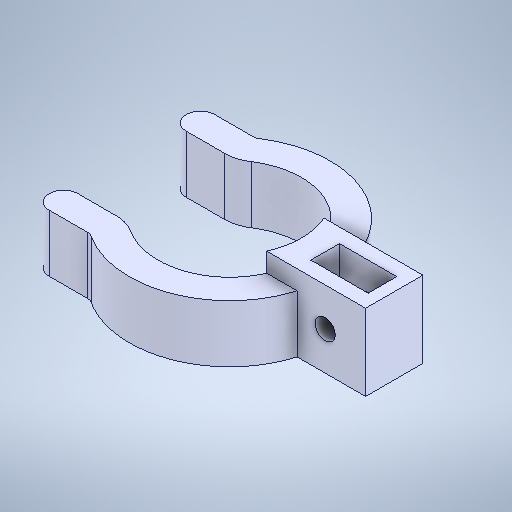
# Autodesk Inventor part: sujetador_marcador_v2
Saved by Autodesk Inventor 2025.2 (Build 292293000, 293)
## iProperties
Created: 2024-08-16
Part Number: sujetador_marcador_v2
Material: Generic
Document SubType Name: Modeling
Designer: cdavi
Density: 1 g/cm^3
Appearance: Default
Sending System: SolidWorks 2024
Last Author: jimen
Last Saved: 2024-10-09
Author: cdavi
Autodesk Inventor part; units mm, degrees
ref_plane "YZ Plane" through (0, 0, 0) normal (1, 0, 0) x (0, 1, 0)
ref_plane "XZ Plane" through (0, 0, 0) normal (0, 1, 0) x (-1, 0, 0)
ref_plane "XY Plane" through (0, 0, 0) normal (0, 0, 1) x (1, 0, 0)
sketch "Sketch1" plane through (0, 0, 0) normal (0, 1, 0) x (-1, 0, 0)
  circle A0 centre (0, 0) radius 7.5
  circle A1 centre (0, 0) radius 10.5
  line L0 (0, 0) -> (5.6818, 8.8299) construction
  line L1 (0, 0) -> (0, 10.5)
  line L2 (6.222, 8.6714) -> (10.222, 8.6714)
  arc A2 (5.6818, 8.8299) -> (6.222, 8.6714) centre (6.222, 9.6714) ccw
  line L3 (6.222, 5.6714) -> (10.222, 5.6714)
  arc A3 (4.0584, 6.3071) -> (6.222, 5.6714) centre (6.222, 9.6714) ccw
  line L4 (10.222, 8.6714) -> (10.222, 5.6714) construction
  arc A4 (10.222, 5.6714) -> (10.222, 8.6714) centre (10.222, 7.1714) ccw
  line L5 (0, 0) -> (7.5, 0)
  line L6 (6.222, -8.6714) -> (10.222, -8.6714)
  arc A5 (6.222, -8.6714) -> (5.6818, -8.8299) centre (6.222, -9.6714) ccw
  line L7 (6.222, -5.6714) -> (10.222, -5.6714)
  arc A6 (6.222, -5.6714) -> (4.0584, -6.3071) centre (6.222, -9.6714) ccw
  arc A7 (10.222, -8.6714) -> (10.222, -5.6714) centre (10.222, -7.1714) ccw
  point P0 (4.0584, -6.3071)
  dimension "d0" = 15
  dimension "d1" = 3
  dimension "d2" = 32.76
  dimension "d3" = 1
  dimension "d4" = 3
  dimension "d5" = 4
  dimension "d6" = 6.222
  dimension "d7" = 4
  constraints: 16 end point, 16 point on circle, 9 symmetric about line, 8 centre point, 3 horizontal, 2 coincident, 2 tangent, 2 vertical, 1 midpoint, 1 point on line, 1 vertical alignment, 3 other
  measures "d0" diameter of A0
  measures "d1" radial gap between concentric circles of A1 A0
  measures "d2" angle of L1 L0
  measures "d3" radius of A2
  measures "d4" distance between parallel lines of L3 L2
  measures "d5" radius of A3
  measures "d6" distance from line of L1 L2.start
  measures "d7" distance of L2.start L2.end
extrude "Extrusion1" add sketch "Sketch1" along normal blind 6 contours A0 L1 A1 L3 A3 | A6 L7 A1 L1 A0 | A1 A2 L2 A4 L3 | L7 A7 L6 A5 A1
sketch "Sketch2" plane through (0, 0, 0) normal (0, -1, 0) x (1, 0, 0)
  arc A0 (-5.6818, -8.8299) -> (-5.6818, 8.8299) centre (0, 0) ccw projected
  line L0 (6.8739, 3) -> (17.234, 3)
  line L1 (17.234, 3) -> (17.234, -3)
  line L2 (17.234, -3) -> (6.8739, -3)
  line L3 (6.8739, -3) -> (6.8739, 3)
  line L4 (10.5, 0) -> (17.234, 0)
  arc A1 (-4.0584, -6.3071) -> (-4.0584, 6.3071) centre (0, 0) ccw projected
  circle A2 centre (0, 0) radius 7.5 projected
  arc A3 (-5.6818, -8.8299) -> (-5.6818, 8.8299) centre (0, 0) ccw projected
  line L5 (10, -1.5) -> (16, -1.5)
  line L6 (16, -1.5) -> (16, 1.5)
  line L7 (16, 1.5) -> (10, 1.5)
  line L8 (10, 1.5) -> (10, -1.5)
  arc A4 (-4.0584, -6.3071) -> (-4.0584, 6.3071) centre (0, 0) ccw projected
  point P0 (10.0623, 3)
  point P1 (13.867, 0)
  point P2 (6.8739, -3)
  point P3 (10, 0)
  point P4 (7.5, 0)
  dimension "d11" = 6
  dimension "d12" = 1.234
  dimension "d14" = 6
  dimension "d20" = 2.5
  dimension "d25" = 3
  constraints: 18 end point, 4 midpoint, 4 parallel, 4 point on circle, 3 perpendicular, 2 horizontal, 1 point on line, 1 other
  measures "d11" distance of L0.end L1.end
  measures "d12" distance between parallel lines of L1 L6
  measures "d14" distance between parallel lines of L8 L6
  measures "d20" distance of point (10, 0) point (7.5, 0)
  measures "d25" distance between parallel lines of L7 L5
extrude "Extrusion2" add sketch "Sketch2" against normal blind 8 contours L2 A1 L0 A0 L7 L8 L5 | A0 L5 L6 L4 L1 L2 | L5 L8 L7 A0 | A0 L4 L6 L5 | A0 L7 L6 L4 | L4 L6 L7 A0 L0 L1
ref_plane "Work Plane1" through (0, 0.5, 0) normal (0, -1, 0) x (1, 0, 0)
extrude "Extrusion3" cut sketch "Sketch2" against normal blind 8 from surface at -0.5 contours L5 L8 L7 A0 | A0 L4 L6 L5 | A0 L7 L6 L4
sketch "Sketch3" plane through (10.0623, 0, 3) normal (0, 0, 1) x (1, 0, 0)
  circle A0 centre (2.9377, 4) radius 1.05
  line L0 (5.9377, 0.5) -> (-0.0623, 0.5) projected
  point P0 (-10.0623, 0)
  point P1 (2.9377, 0.5)
  dimension "d21" = 2.1
  dimension "d22" = 3.5
  constraints: 1 centre point, 1 midpoint, 1 vertical alignment
  measures "d21" diameter of A0
  measures "d22" distance of point (2.938, 0.5) A0.centre
extrude "Extrusion4" cut sketch "Sketch3" against normal through all
body "Solid2"
